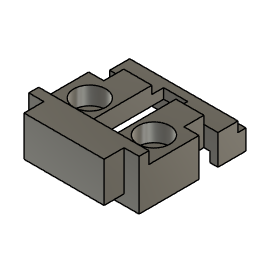
Peca Porta Buinho v18 (Autodesk Fusion 360 design; units mm, degrees)
Autodesk Fusion 360 part; units mm, degrees
sketch "Sketch1" plane through (0, 0, 0) normal (0, 0, 1) x (1, 0, 0) in component "PecaPorta"
  line L0 (-37.704, -20.0025) -> (-33.9529, -19.9954)
  line L1 (-33.9529, -19.9954) -> (-33.9623, -14.9954)
  line L2 (-33.9623, -14.9954) -> (-37.4642, -15.002)
  line L3 (-37.4642, -15.002) -> (-37.4736, -10.0032)
  line L4 (-37.704, -20.0025) -> (-37.6758, -35.0025)
  line L5 (-10.4698, -9.9525) -> (-10.4604, -14.9513)
  line L6 (-10.1737, -34.9508) -> (-10.2018, -19.9508)
  line L7 (-10.2018, -19.9508) -> (-13.9529, -19.9579)
  line L8 (-13.9529, -19.9579) -> (-13.9623, -14.9579)
  line L9 (-10.4604, -14.9513) -> (-13.9623, -14.9579)
  line L10 (-26.9294, -32.5252) -> (-20.9294, -32.514)
  line L11 (-20.9294, -32.514) -> (-20.9679, -12.014)
  line L12 (-20.9679, -12.014) -> (-26.9679, -12.0253)
  line L13 (-26.9679, -12.0253) -> (-26.9294, -32.5252)
  circle A0 centre (-31.9407, -25.5003) radius 4
  circle A1 centre (-15.9407, -25.4703) radius 4
  line L14 (-33.9154, -39.9508) -> (-13.9154, -39.9508)
  line L15 (-33.9154, -39.9508) -> (-33.9247, -34.9954)
  line L16 (-13.9154, -39.9508) -> (-13.9248, -34.9579)
  line L17 (-10.4698, -9.9525) -> (-37.4736, -10.0032)
  circle A2 centre (-31.9407, -25.5003) radius 2.25
  circle A3 centre (-15.9407, -25.4703) radius 2.25
  line L18 (-10.4736, -7.9525) -> (-10.4698, -9.9525)
  line L19 (-10.4736, -7.9525) -> (-37.4736, -8.0032)
  line L20 (-37.4736, -8.0032) -> (-37.4736, -10.0032)
  line L21 (-37.6758, -35.0025) -> (-33.9247, -34.9954)
  line L22 (-13.9248, -34.9579) -> (-10.1737, -34.9508)
  line L23 (-13.9248, -34.9579) -> (-33.9247, -34.9954)
  line L24 (-12.1877, -32.9568) -> (-12.1991, -26.8848)
  line L25 (-12.2045, -24.0418) -> (-12.2084, -21.9579)
  line L26 (-12.2084, -21.9579) -> (-14.0206, -21.9613)
  line L27 (-15.9576, -12.9546) -> (-15.9416, -21.4703)
  line L28 (-15.9576, -12.9546) -> (-12.4668, -12.9481)
  line L29 (-12.4668, -12.9481) -> (-12.4724, -9.9562)
  line L30 (-12.1877, -32.9568) -> (-35.6814, -33.0009)
  line L31 (-35.6814, -33.0009) -> (-35.6929, -26.8864)
  line L32 (-35.6981, -24.1284) -> (-35.7021, -21.9994)
  line L33 (-33.8756, -21.9994) -> (-35.7021, -21.9994)
  line L34 (-31.9576, -21.5004) -> (-31.9736, -12.9987)
  line L35 (-31.9736, -12.9987) -> (-35.4689, -12.9987)
  line L36 (-35.4689, -12.9987) -> (-35.4745, -9.9994)
  line L37 (-13.9623, -14.9579) -> (-20.9623, -14.971)
  line L38 (-33.9623, -14.9954) -> (-26.9623, -14.9823)
  dimension "d28" = 20
  dimension "d40" = 27
  constraint perpendicular L6 L7
  constraint perpendicular L7 L8
  constraint equal L0 L7
  constraint equal L2 L9
  constraint equal L1 L8
  constraint equal L4 L6
  constraint perpendicular L10 L11
  constraint parallel L10 L12
  constraint parallel L11 L13
  constraint horizontal L14
  constraint perpendicular L3 L17
  constraint perpendicular L5 L9
  constraint perpendicular L8 L9
  constraint perpendicular L2 L3
  constraint perpendicular L1 L2
  constraint perpendicular L0 L1
  constraint perpendicular L17 L18
  constraint perpendicular L3 L19
  constraint vertical L20
  constraint parallel L21 L22
  constraint parallel L21 L23
  constraint coincident A1 L24.end
  constraint coincident A1 L25.start
  constraint parallel L24 L25
  constraint coincident A1 L26.end
  constraint perpendicular L25 L26
  constraint coincident A1 L27.end
  constraint perpendicular L27 L28
  constraint coincident L17 L29.end
  constraint perpendicular L17 L29
  constraint perpendicular L24 L30
  constraint coincident A0 L31.end
  constraint perpendicular L30 L31
  constraint coincident A0 L32.start
  constraint coincident A0 L33.start
  constraint horizontal L33
  constraint coincident A0 L34.start
  constraint coincident L17 L36.end
  constraint perpendicular L17 L36
  constraint coincident L11 L37.end
  constraint perpendicular L11 L37
  constraint coincident L13 L38.end
  constraint perpendicular L13 L38
  measures "d28" distance of L14.start L14.end
  measures "d40" horizontal distance of L18.start L19.end
extrude "Extrude7" add sketch "Sketch1" along normal blind 2.5 contours L0 L1 L4 L6 L7 L8 A0 A1 L21 L22 L23 L24 L25 L26 L27 L30 L31 L32 L33 L34 L37 L38 | L2 L3 L17 L34 L35 L36 L38 | L14 L15 L16 L23 | L10 L11 L13 A0 A1 L24 L27 L30 L31 L34 L37 L38 | L11 L12 L13 L17 L27 L28 L29 L34 L35 L36 L37 L38 | A0 L32 L33 | L5 L9 L17 L27 L28 L29 L37 | A1 L25 L26
sketch "Sketch3" plane through (0, 0, 2.5) normal (0, 0, 1) x (-1, 0, 0)
  circle A0 centre (31.9407, 25.5003) radius 4
  line L0 (26.9294, 32.5252) -> (26.9679, 12.0253)
  line L1 (26.9679, 12.0253) -> (20.9679, 12.014)
  line L2 (20.9679, 12.014) -> (20.9294, 32.514)
  line L3 (20.9294, 32.514) -> (26.9294, 32.5252)
  circle A1 centre (15.9407, 25.4703) radius 4
  line L4 (33.9154, 39.9508) -> (13.9154, 39.9508)
  line L5 (13.9154, 39.9508) -> (13.9248, 34.9579)
  line L6 (13.9248, 34.9579) -> (10.1737, 34.9508)
  line L7 (10.1737, 34.9508) -> (10.2018, 19.9508)
  line L8 (10.2018, 19.9508) -> (13.9529, 19.9579)
  line L9 (13.9529, 19.9579) -> (13.9623, 14.9579)
  line L10 (13.9623, 14.9579) -> (10.4604, 14.9513)
  line L11 (10.4604, 14.9513) -> (10.4698, 9.9525)
  line L12 (10.4698, 9.9525) -> (37.4736, 10.0032)
  line L13 (37.4736, 10.0032) -> (37.4642, 15.002)
  line L14 (37.4642, 15.002) -> (33.9623, 14.9954)
  line L15 (33.9623, 14.9954) -> (33.9529, 19.9954)
  line L16 (33.9529, 19.9954) -> (37.704, 20.0025)
  line L17 (37.704, 20.0025) -> (37.6758, 35.0025)
  line L18 (37.6758, 35.0025) -> (33.9247, 34.9954)
  line L19 (33.9247, 34.9954) -> (33.9154, 39.9508)
  line L20 (13.9623, 14.9579) -> (20.9623, 14.971)
  line L21 (33.9623, 14.9954) -> (26.9623, 14.9823)
  point P0 (20.9623, 14.971)
  point P1 (26.9623, 14.9823)
  constraint coincident L9.end L10.start
  constraint coincident P0 L20.end
  constraint coincident L14.end L15.start
  constraint coincident P1 L21.end
extrude "Extrude8" add sketch "Sketch3" along normal blind 2 contours L0 L2 L3 L4 L5 L6 L7 L8 L9 L15 L16 L17 L18 L19 L20 L21
extrude "Extrude9" add sketch "Sketch1" against normal blind 2.5 contours L0 L1 L4 L6 L7 L8 A0 A1 L21 L22 L23 L24 L25 L26 L27 L30 L31 L32 L33 L34 L37 L38 | L2 L3 L17 L34 L35 L36 L38 | L14 L15 L16 L23 | L17 L18 L19 L20 | A0 | A0 L32 L33 | L5 L9 L17 L27 L28 L29 L37 | A1 | A1 L25 L26
sketch "Sketch4" plane through (0, 0, -2.5) normal (0, 0, -1) x (1, 0, 0)
  circle A0 centre (-31.9407, 25.5003) radius 2.25
  line L0 (-12.1877, 32.9568) -> (-12.1991, 26.8848)
  arc A1 (-12.1991, 26.8848) -> (-15.9416, 21.4703) centre (-15.9407, 25.4703) ccw
  line L1 (-15.9416, 21.4703) -> (-15.9576, 12.9546)
  line L2 (-15.9576, 12.9546) -> (-12.4668, 12.9481)
  line L3 (-12.4668, 12.9481) -> (-12.4724, 9.9562)
  line L4 (-12.4724, 9.9562) -> (-35.4745, 9.9994)
  line L5 (-35.4745, 9.9994) -> (-35.4689, 12.9987)
  line L6 (-35.4689, 12.9987) -> (-31.9736, 12.9987)
  line L7 (-31.9736, 12.9987) -> (-31.9576, 21.5004)
  arc A2 (-31.9576, 21.5004) -> (-35.6929, 26.8864) centre (-31.9407, 25.5003) ccw
  line L8 (-35.6929, 26.8864) -> (-35.6814, 33.0009)
  line L9 (-35.6814, 33.0009) -> (-12.1877, 32.9568)
  circle A3 centre (-15.9407, 25.4703) radius 2.25
  line L10 (-13.9154, 39.9508) -> (-33.9154, 39.9508)
  line L11 (-33.9154, 39.9508) -> (-33.9247, 34.9954)
  line L12 (-33.9247, 34.9954) -> (-37.6758, 35.0025)
  line L13 (-37.6758, 35.0025) -> (-37.704, 20.0025)
  line L14 (-37.704, 20.0025) -> (-33.9529, 19.9954)
  line L15 (-33.9529, 19.9954) -> (-33.9623, 14.9954)
  line L16 (-33.9623, 14.9954) -> (-37.4642, 15.002)
  line L17 (-37.4642, 15.002) -> (-37.4736, 10.0032)
  line L18 (-37.4736, 10.0032) -> (-37.4736, 8.0032)
  line L19 (-37.4736, 8.0032) -> (-10.4736, 7.9525)
  line L20 (-10.4736, 7.9525) -> (-10.4604, 14.9513)
  line L21 (-10.4604, 14.9513) -> (-13.9623, 14.9579)
  line L22 (-13.9623, 14.9579) -> (-13.9529, 19.9579)
  line L23 (-13.9529, 19.9579) -> (-10.2018, 19.9508)
  line L24 (-10.2018, 19.9508) -> (-10.1737, 34.9508)
  line L25 (-10.1737, 34.9508) -> (-13.9248, 34.9579)
  line L26 (-13.9248, 34.9579) -> (-13.9154, 39.9508)
  line L27 (-35.4689, 12.9987) -> (-35.4651, 14.9983)
  line L28 (-33.9247, 34.9954) -> (-13.9248, 34.9579)
  line L29 (-12.4668, 12.9481) -> (-12.463, 14.9551)
  circle A4 centre (-15.9407, 25.4703) radius 4
  circle A5 centre (-31.9407, 25.5003) radius 4
  line L30 (-15.9416, 21.4703) -> (-12.2093, 21.4694)
  line L31 (-12.2093, 21.4694) -> (-12.2122, 19.9546)
  line L32 (-31.9576, 21.5004) -> (-35.703, 21.5162)
  line L33 (-35.703, 21.5162) -> (-35.7058, 19.9987)
  constraint coincident L5.end L6.start
  constraint coincident L16 L27.end
  constraint perpendicular L16 L27
  constraint coincident L11.end L12.start
  constraint coincident L25.end L26.start
  constraint coincident L2.end L3.start
  constraint coincident L21 L29.end
  constraint perpendicular L21 L29
  constraint concentric A1 A4
  constraint coincident A1.end A4
  constraint concentric A0 A5
  constraint coincident L7.end A5
  constraint coincident A1.end L1.start
  constraint tangent A4 L30
  constraint coincident L23 L31.end
  constraint perpendicular L23 L31
  constraint coincident L7.end A2.start
  constraint tangent A5 L32
  constraint coincident L14 L33.end
  constraint perpendicular L14 L33
extrude "Extrude10" add sketch "Sketch4" along normal blind 2.5 contours L0 L8 L9 L12 L13 L14 L23 L24 L25 L28 A4 A5 L30 L31 L32 L33 | A1 A4 | A2 A5 | L3 L4 L5 L16 L17 L18 L19 L20 L21 L27 L29
sketch "Sketch5" plane through (0, 0, 4.5) normal (0, 0, 1) x (-1, 0, 0)
  circle A0 centre (15.9407, 25.4703) radius 4
  circle A1 centre (31.9407, 25.5003) radius 4
  line L0 (33.9529, 19.9954) -> (37.704, 20.0025)
  line L1 (37.704, 20.0025) -> (37.6758, 35.0025)
  line L2 (37.6758, 35.0025) -> (33.9247, 34.9954)
  line L3 (33.9247, 34.9954) -> (33.9154, 39.9508)
  line L4 (33.9154, 39.9508) -> (13.9154, 39.9508)
  line L5 (13.9154, 39.9508) -> (13.9248, 34.9579)
  line L6 (13.9248, 34.9579) -> (10.1737, 34.9508)
  line L7 (10.1737, 34.9508) -> (10.2018, 19.9508)
  line L8 (10.2018, 19.9508) -> (13.9529, 19.9579)
  line L9 (13.9529, 19.9579) -> (13.9623, 14.9579)
  line L10 (13.9623, 14.9579) -> (20.9623, 14.971)
  line L11 (20.9623, 14.971) -> (20.9294, 32.514)
  line L12 (20.9294, 32.514) -> (26.9294, 32.5252)
  line L13 (26.9294, 32.5252) -> (26.9623, 14.9823)
  line L14 (26.9623, 14.9823) -> (33.9623, 14.9954)
  line L15 (33.9623, 14.9954) -> (33.9529, 19.9954)
  line L16 (20.9294, 32.514) -> (10.1783, 32.4938)
  line L17 (26.9294, 32.5252) -> (37.6805, 32.5454)
  constraint coincident L11.end L12.start
  constraint coincident L7 L16.end
  constraint perpendicular L7 L16
  constraint coincident L12.end L13.start
  constraint coincident L1 L17.end
  constraint perpendicular L1 L17
extrude "Extrude11" add sketch "Sketch5" along normal blind 3 contours L1 L2 L3 L4 L5 L6 L7 L12 L16 L17
component "PecaPorta" placed x (1, 0, 0) y (0, 1, 0) z (0, 0, 1) at (0, 0, 0)
named bodies: "peca_porta"
